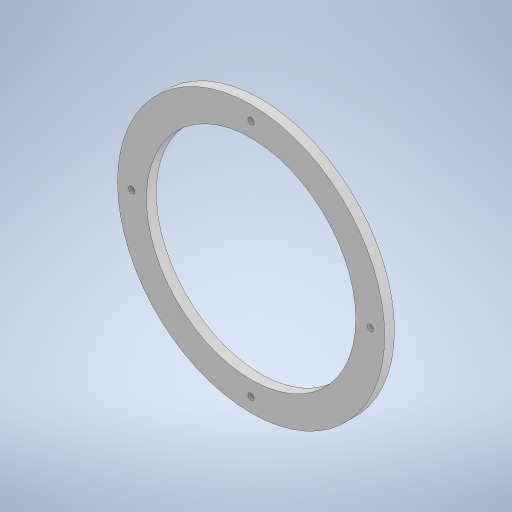
# Autodesk Inventor part: 아크릴 빛번짐 고정용
Saved by Autodesk Inventor 2023 (Build 270158000, 158)
## iProperties
Created: 2022-06-05
Part Number: 아크릴 빛번짐 고정용
Material: 일반
Document SubType Name: Modeling
Designer: fly01
Density: 1 g/cm^3
Appearance: 기본값
Author: fly01
Autodesk Inventor part; units mm, degrees
ref_plane "YZ Plane" through (0, 0, 0) normal (1, 0, 0) x (0, 1, 0)
ref_plane "XZ Plane" through (0, 0, 0) normal (0, 1, 0) x (-1, 0, 0)
ref_plane "XY Plane" through (0, 0, 0) normal (0, 0, 1) x (1, 0, 0)
sketch "스케치1" plane through (0, 0, 0) normal (0, 0, 1) x (1, 0, 0)
  circle A0 centre (0, 0) radius 68.25
  circle A1 centre (0, 0) radius 53.5
  circle A2 centre (0, 0) radius 61 construction
  circle A3 centre (0, 61) radius 1.6
  circle A4 centre (-61, 0) radius 1.6
  circle A5 centre (0, -61) radius 1.6
  circle A6 centre (61, 0) radius 1.6
  dimension "d2" = 122
  dimension "d0" = 136.5
  dimension "d1" = 107
  dimension "d3" = 3.2
  dimension "d6" = 360
  constraints: 6 centre point, 3 coincident, 1 vertical alignment, 11 other
  measures "d0" diameter of A0
  measures "d1" diameter of A1
  measures "d3" diameter of A3
extrude "돌출1" add sketch "스케치1" along normal blind 5
